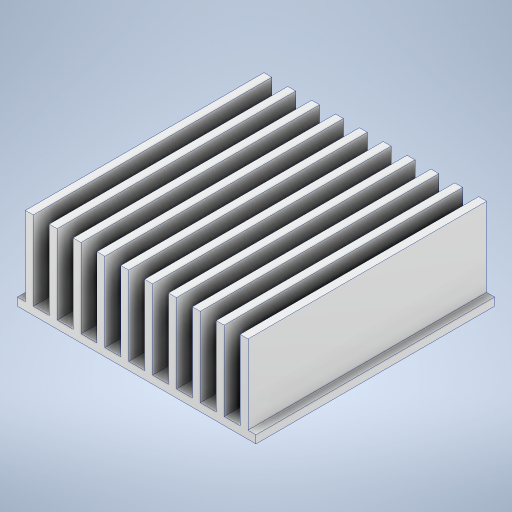
# Autodesk Inventor part: cooler_plate
Saved by Autodesk Inventor 2023 (Build 270158000, 158)
## iProperties
Created: 2023-09-08
Part Number: cooler_plate
Material: Aluminum 6061
Document SubType Name: Modeling
Designer: 310611102
Density: 2.7 g/cm^3
Appearance: Aluminum - Flat
Mass: 10.476 g
Surface Area: 80.7867 cm^2
Volume: 3.88 cm^3
Author: 310611102
Autodesk Inventor part; units mm, degrees
ref_plane "YZ Plane" through (0, 0, 0) normal (1, 0, 0) x (0, 1, 0)
ref_plane "XZ Plane" through (0, 0, 0) normal (0, 1, 0) x (-1, 0, 0)
ref_plane "XY Plane" through (0, 0, 0) normal (0, 0, 1) x (1, 0, 0)
sketch "Sketch1" plane through (0, 0, 0) normal (0, 0, 1) x (1, 0, 0)
  line L0 (-15, 0.5) -> (15, 0.5)
  line L1 (15, 0.5) -> (15, -0.5)
  line L2 (15, -0.5) -> (-15, -0.5)
  line L3 (-15, -0.5) -> (-15, 0.5)
  line L4 (-15, 0.5) -> (15, -0.5) construction
  line L5 (15, 0.5) -> (-15, -0.5) construction
  line L6 (-14, 10.4333) -> (-13, 10.4333)
  line L7 (-13, 10.4333) -> (-13, 0.4333)
  line L8 (-13, 0.4333) -> (-14, 0.4333)
  line L9 (-14, 0.4333) -> (-14, 10.4333)
  line L10 (-14, 10.4333) -> (-13, 0.4333) construction
  line L11 (-13, 10.4333) -> (-14, 0.4333) construction
  line L12 (-11, 10.4333) -> (-10, 10.4333)
  line L13 (-10, 10.4333) -> (-10, 0.4333)
  line L14 (-10, 0.4333) -> (-11, 0.4333)
  line L15 (-11, 0.4333) -> (-11, 10.4333)
  line L16 (-11, 10.4333) -> (-10, 0.4333) construction
  line L17 (-10, 10.4333) -> (-11, 0.4333) construction
  line L18 (-8, 10.4333) -> (-7, 10.4333)
  line L19 (-7, 10.4333) -> (-7, 0.4333)
  line L20 (-7, 0.4333) -> (-8, 0.4333)
  line L21 (-8, 0.4333) -> (-8, 10.4333)
  line L22 (-8, 10.4333) -> (-7, 0.4333) construction
  line L23 (-7, 10.4333) -> (-8, 0.4333) construction
  line L24 (-5, 10.4333) -> (-4, 10.4333)
  line L25 (-4, 10.4333) -> (-4, 0.4333)
  line L26 (-4, 0.4333) -> (-5, 0.4333)
  line L27 (-5, 0.4333) -> (-5, 10.4333)
  line L28 (-5, 10.4333) -> (-4, 0.4333) construction
  line L29 (-4, 10.4333) -> (-5, 0.4333) construction
  line L30 (-2, 10.4333) -> (-1, 10.4333)
  line L31 (-1, 10.4333) -> (-1, 0.4333)
  line L32 (-1, 0.4333) -> (-2, 0.4333)
  line L33 (-2, 0.4333) -> (-2, 10.4333)
  line L34 (-2, 10.4333) -> (-1, 0.4333) construction
  line L35 (-1, 10.4333) -> (-2, 0.4333) construction
  line L36 (1, 10.4333) -> (2, 10.4333)
  line L37 (2, 10.4333) -> (2, 0.4333)
  line L38 (2, 0.4333) -> (1, 0.4333)
  line L39 (1, 0.4333) -> (1, 10.4333)
  line L40 (1, 10.4333) -> (2, 0.4333) construction
  line L41 (2, 10.4333) -> (1, 0.4333) construction
  line L42 (4, 10.4333) -> (5, 10.4333)
  line L43 (5, 10.4333) -> (5, 0.4333)
  line L44 (5, 0.4333) -> (4, 0.4333)
  line L45 (4, 0.4333) -> (4, 10.4333)
  line L46 (4, 10.4333) -> (5, 0.4333) construction
  line L47 (5, 10.4333) -> (4, 0.4333) construction
  line L48 (7, 10.4333) -> (8, 10.4333)
  line L49 (8, 10.4333) -> (8, 0.4333)
  line L50 (8, 0.4333) -> (7, 0.4333)
  line L51 (7, 0.4333) -> (7, 10.4333)
  line L52 (7, 10.4333) -> (8, 0.4333) construction
  line L53 (8, 10.4333) -> (7, 0.4333) construction
  line L54 (10, 10.4333) -> (11, 10.4333)
  line L55 (11, 10.4333) -> (11, 0.4333)
  line L56 (11, 0.4333) -> (10, 0.4333)
  line L57 (10, 0.4333) -> (10, 10.4333)
  line L58 (10, 10.4333) -> (11, 0.4333) construction
  line L59 (11, 10.4333) -> (10, 0.4333) construction
  line L60 (13, 10.4333) -> (14, 10.4333)
  line L61 (14, 10.4333) -> (14, 0.4333)
  line L62 (14, 0.4333) -> (13, 0.4333)
  line L63 (13, 0.4333) -> (13, 10.4333)
  line L64 (13, 10.4333) -> (14, 0.4333) construction
  line L65 (14, 10.4333) -> (13, 0.4333) construction
  point P0 (0, 0)
  point P1 (-13.5, 5.4333)
  point P2 (-12, 0.5)
  point P3 (-10.5, 5.4333)
  point P4 (-9, 0.5)
  point P5 (-7.5, 5.4333)
  point P6 (-6, 0.5)
  point P7 (-4.5, 5.4333)
  point P8 (-3, 0.5)
  point P9 (-1.5, 5.4333)
  point P10 (0, 0.5)
  point P11 (1.5, 5.4333)
  point P12 (3, 0.5)
  point P13 (4.5, 5.4333)
  point P14 (6, 0.5)
  point P15 (7.5, 5.4333)
  point P16 (9, 0.5)
  point P17 (10.5, 5.4333)
  point P18 (12, 0.5)
  point P19 (13.5, 5.4333)
  point P20 (13, 0.5)
  point P21 (11, 0.5)
  point P22 (10, 0.5)
  point P23 (8, 0.5)
  point P24 (7, 0.5)
  point P25 (5, 0.5)
  point P26 (4, 0.5)
  point P27 (2, 0.5)
  point P28 (1, 0.5)
  point P29 (-1, 0.5)
  point P30 (-2, 0.5)
  point P31 (-4, 0.5)
  point P32 (-5, 0.5)
  point P33 (-7, 0.5)
  point P34 (-8, 0.5)
  point P35 (-10, 0.5)
  point P36 (-11, 0.5)
  point P37 (-13, 0.5)
  point P38 (14, 0.5)
  point P39 (-14, 0.5)
  dimension "d0" = 1
  dimension "d1" = 30
  dimension "d2" = 1
  dimension "d3" = 10
  dimension "d6" = 3
  dimension "d13" = 1
  dimension "d14" = 1
  constraints: 130 end point, 4 midpoint, 3 horizontal, 3 parallel, 1 collinear, 1 perpendicular, 1 point on line, 1 vertical, 110 other
  measures "d0" distance of L1.start L1.end
  measures "d1" distance of L1.end L2.end
  measures "d2" distance of L6.start L6.end
  measures "d3" distance of L8.end L6.start
  measures "d6" distance of L3.end point (-12, 0.5)
  measures "d13" distance between parallel lines of L3 L9
  measures "d14" distance between parallel lines of L1 L61
extrude "Extrusion1" add sketch "Sketch1" along normal blind 30
body "Solid1"
